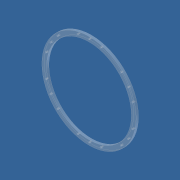
# Autodesk Inventor part: JF-AT-TM0008
Saved by Autodesk Inventor 2012 SP2 (Build 160219200, 219)
## iProperties
Created: 2010-04-06
Part Number: JF-AT-TM0008
Document SubType Name: Modeling
Designer: Osborne J.
Density: 0.66 g/cm^3
Material: Acrylic, Clear
Mass: 458.7 g
Surface Area: 1641.73 cm^2
Volume: 695 cm^3
Description: 16 inch ball treadmill top ring v2
Title: 16 inch ball treadmill top ring v2
Author: Osborne J.
Autodesk Inventor part; units mm, degrees
ref_plane "YZ Plane" through (0, 0, 0) normal (1, 0, 0) x (0, 1, 0)
ref_plane "XZ Plane" through (0, 0, 0) normal (0, 1, 0) x (-1, 0, 0)
ref_plane "XY Plane" through (0, 0, 0) normal (0, 0, 1) x (1, 0, 0)
sketch "Sketch1" plane through (0, 0, 0) normal (0, 0, 1) x (1, 0, 0)
  circle A0 centre (0, 0) radius 254
  circle A1 centre (0, 0) radius 228.6
  line L0 (0, 0) -> (0, 394.3649)
  line L1 (0, 0) -> (92.6141, 345.6404)
  line L2 (0, 0) -> (-94.6299, 353.1634)
  circle A2 centre (0, 0) radius 241.3
  point P0 (-62.453, 233.0779)
  point P1 (0, 241.3)
  point P2 (62.453, 233.0779)
  point P3 (-233.0779, 62.453)
  point P4 (-208.9719, 120.65)
  point P5 (-170.6249, 170.6249)
  point P6 (-170.6249, -170.6249)
  point P7 (-208.9719, -120.65)
  point P8 (-233.0779, -62.453)
  point P9 (62.453, -233.0779)
  point P10 (0, -241.3)
  point P11 (-62.453, -233.0779)
  point P12 (233.0779, -62.453)
  point P13 (208.9719, -120.65)
  point P14 (170.6249, -170.6249)
  point P15 (170.6249, 170.6249)
  point P16 (208.9719, 120.65)
  point P17 (233.0779, 62.453)
  dimension "d0" = 508
  dimension "d1" = 457.2
  dimension "d4" = 30
  dimension "d5" = 15
  dimension "d6" = 482.6
  dimension "d9" = 360
  constraints: 6 end point, 3 centre point, 3 coincident, 3 point on circle, 3 point on line, 1 vertical, 19 other
  measures "d0" diameter of A0
  measures "d1" diameter of A1
  measures "d4" angle of L1 L2
  measures "d5" angle of L0 L2
  measures "d6" diameter of A2
extrude "Extrusion1" add sketch "Sketch1" along normal blind 12.7 contours A0 L2 A2 L1 | L1 A2 L0 A0 | A0 L0 A2 L2 | A2 L2 A1 L1 | L1 A1 L0 A2 | A2 L0 A1 L2
hole "Hole1" at (-62.453, 233.0779, 0) at (0, 241.3, 0) at (62.453, 233.0779, 0) at (-170.6249, 170.6249, 0) at (-208.9719, 120.65, 0) at (-233.0779, 62.453, 0) at (-233.0779, -62.453, 0) at (-208.9719, -120.65, 0) at (-170.6249, -170.6249, 0) at (-62.453, -233.0779, 0) at (0, -241.3, 0) at (62.453, -233.0779, 0) at (170.6249, -170.6249, 0) at (208.9719, -120.65, 0) at (233.0779, -62.453, 0) at (233.0779, 62.453, 0) at (208.9719, 120.65, 0) at (170.6249, 170.6249, 0) direction (0, 0, 1) diameter 7.1374 end through all
body "Solid1"
